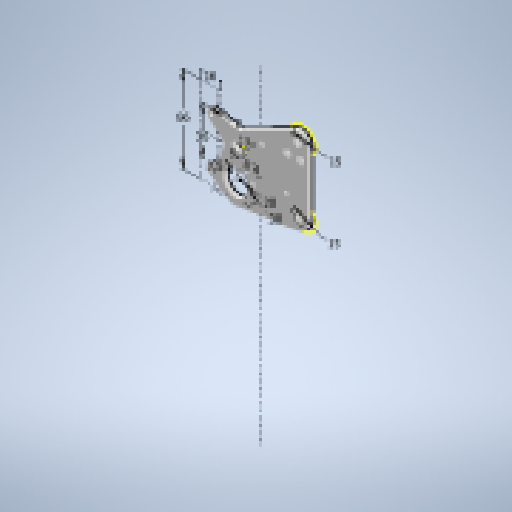
# Autodesk Inventor part: plate_3
Saved by Autodesk Inventor 2024 (Build 280153000, 153)
## iProperties
Created: 2026-02-08
Part Number: plate_3
Material: Generic
Document SubType Name: Modeling
Designer: SEMEN
Density: 1 g/cm^3
Appearance: Default
Author: SEMEN
Autodesk Inventor part; units mm, degrees
ref_plane "YZ Plane" through (0, 0, 0) normal (1, 0, 0) x (0, 1, 0)
ref_plane "XZ Plane" through (0, 0, 0) normal (0, 1, 0) x (-1, 0, 0)
ref_plane "XY Plane" through (0, 0, 0) normal (0, 0, 1) x (1, 0, 0)
sketch "Sketch1" plane through (0, 0, 0) normal (0, 0, 1) x (1, 0, 0)
  circle A0 centre (57.407, 53.064) radius 2.5 projected
  circle A1 centre (57.407, 53.064) radius 10 projected
  circle A2 centre (13.407, 27.6606) radius 2.5 projected
  circle A3 centre (13.407, 27.6606) radius 10 projected
  circle A4 centre (57.407, 2.2572) radius 2.5 projected
  circle A5 centre (57.407, 2.2572) radius 10 projected
  line L0 (25.407, -164.9104) -> (25.407, 85.0896) construction
  arc A6 (64.907, 53.064) -> (53.9811, 59.7359) centre (57.407, 53.064) ccw
  arc A7 (58.5116, -5.161) -> (64.907, 2.2572) centre (57.407, 2.2572) ccw
  line L1 (10.407, 27.6606) -> (16.407, 27.6606) construction
  line L2 (10.407, 25.0106) -> (16.407, 25.0106)
  line L3 (16.407, 30.3106) -> (10.407, 30.3106)
  arc A8 (10.407, 30.3106) -> (10.407, 25.0106) centre (10.407, 27.6606) ccw
  arc A9 (16.407, 25.0106) -> (16.407, 30.3106) centre (16.407, 27.6606) ccw
  circle A10 centre (10.407, 2.8412) radius 10
  arc A11 (-3.8238, 7.5832) -> (12.6162, -11.9952) centre (10.407, 2.8412) ccw
  line L4 (12.6162, -11.9952) -> (58.5116, -5.161)
  line L5 (53.9811, 59.7359) -> (8.8392, 36.5564)
  line L6 (64.907, 2.2572) -> (64.907, 53.064)
  line L7 (3.9198, 30.8219) -> (-3.8238, 7.5832)
  line L8 (-3.8238, 7.5832) -> (-11.5466, -15.5932) construction
  line L9 (12.6162, -11.9952) -> (-11.5466, -15.5932) construction
  line L10 (-11.5466, -15.5932) -> (31.917, 20.9033) construction
  line L11 (-8.093, 51.8526) -> (-8.093, -0.1388) construction
  circle A12 centre (-8.093, 38.8412) radius 3.5 construction
  circle A13 centre (-8.093, 2.8412) radius 3.5 construction
  line L12 (-20.593, 53.8412) -> (-4.593, 53.8412) construction
  line L13 (-4.593, 53.8412) -> (-4.593, -12.1588) construction
  line L14 (-4.593, -12.1588) -> (-20.593, -12.1588) construction
  line L15 (-20.593, -12.1588) -> (-20.593, 53.8412) construction
  line L16 (-20.593, 20.8412) -> (-4.593, 20.8412) construction
  line L17 (-2.413, 11.817) -> (-10.2687, 5.5829)
  line L18 (-10.2687, 0.0996) -> (1.0826, -8.9085)
  arc A14 (-4.593, -1.7035) -> (-4.0348, -1.2128) centre (-8.093, 2.8412) ccw
  arc A15 (-10.2687, 5.5829) -> (-10.2687, 0.0996) centre (-8.093, 2.8412) ccw
  line L19 (1.8905, 24.7319) -> (-10.4816, 36.2829)
  line L20 (-7.3703, 42.2658) -> (11.9978, 38.1783)
  arc A16 (-7.3703, 42.2658) -> (-10.4816, 36.2829) centre (-8.093, 38.8412) ccw
  point P0 (18.407, 14.782)
  point P1 (23.5514, 8.6555)
  dimension "d52" = 15
  dimension "d53" = 15
  dimension "d54" = 3
  dimension "d55" = 5.3
  dimension "d56" = 20
  dimension "d57" = 30
  dimension "d58" = 4
  dimension "d59" = 8
  dimension "d93" = 7
  dimension "d94" = 7
  dimension "d95" = 36
  dimension "d96" = 16
  dimension "d97" = 66
  dimension "d99" = 3.5
  constraints: 44 end point, 25 tangent, 20 point on circle, 11 centre point, 7 coincident, 7 point on line, 3 midpoint, 3 parallel, 2 collinear, 2 horizontal, 2 symmetric about line, 2 vertical, 1 concentric, 1 perpendicular, 2 other
  measures "d52" diameter of A6
  measures "d53" diameter of A7
  measures "d54" distance of A3.centre L1.end
  measures "d55" diameter of A9
  measures "d56" diameter of A10
  measures "d57" diameter of A11
  measures "d58" distance from line of L10 point (18.407, 14.782)
  measures "d59" horizontal distance of A10.centre point (18.407, 14.782)
  measures "d93" diameter of A12
  measures "d94" diameter of A13
  measures "d95" distance of point (-8.093, 2.841) point (-8.093, 38.841)
  measures "d96" distance of L12.start L12.end
  measures "d97" distance of L14.end L12.start
  measures "d99" radius of A15
extrude "Extrusion1" add sketch "Sketch1" along normal blind 4 contours A0 | L5 A6 L6 A1 | A1 L6 A5 L4 A11 L7 A3 L5 | L5 A3 L7 L19 A16 L20 | L6 A7 L4 A5 | A3 | L18 A15 L17 L7 A11 | A4 picked at (52.4239, 56.8921) picked at (55.6672, -3.7922)
sketch "Sketch2" plane through (0, 0, 4) normal (0, 0, 1) x (1, 0, 0)
  circle A0 centre (13.407, 27.6606) radius 2.5 projected
  circle A1 centre (57.407, 2.2572) radius 2.5 projected
  circle A2 centre (57.407, 53.064) radius 2.5 projected
  line L0 (10.407, 27.6606) -> (16.407, 27.6606) construction
  line L1 (10.407, 24.9106) -> (16.407, 24.9106)
  line L2 (16.407, 30.4106) -> (10.407, 30.4106)
  arc A3 (10.407, 30.4106) -> (10.407, 24.9106) centre (10.407, 27.6606) ccw
  arc A4 (16.407, 24.9106) -> (16.407, 30.4106) centre (16.407, 27.6606) ccw
  point P0 (0, 0)
  dimension "d25" = 3
  dimension "d26" = 5.5
  constraints: 8 end point, 4 point on circle, 4 tangent, 2 centre point, 1 horizontal, 1 midpoint, 1 parallel
  measures "d25" distance of A0.centre L0.end
  measures "d26" diameter of A4
hole "Hole2" at (57.407, 53.064, 4) at (57.407, 2.2572, 4) direction (0, 0, -1) diameter 5.5 end through all clearance for "Countersunk Head GOST 12876-67" size "M5" standard "GOST"
hole "Hole4" at (18.407, 14.782, 0) at (23.5514, 8.6555, 0) direction (0, 0, 1) diameter 3 end through all
sketch "Sketch6" plane through (0, 0, 0) normal (0, 0, -1) x (-1, 0, 0)
  circle A0 centre (-49.2903, 15.4803) radius 1.7 projected
  circle A1 centre (-30.2236, 38.1868) radius 1.7 projected
  point P0 (0, 0)
hole "Hole6" at (49.2903, 15.4803, 0) at (30.2236, 38.1868, 0) direction (0, 0, 1) diameter 3.4 end through all countersink diameter 6.6 countersink angle 90 clearance for "Countersunk Head GOST 12876-67" size "M3" standard "GOST"
sketch "Sketch7" plane through (0, 0, 4) normal (0, 0, 1) x (1, 0, 0)
  point P0 (0, 0)
  point P1 (49.6217, 42.3118)
  point P2 (59.6217, 42.3118)
hole "Hole7" at (59.6217, 42.3118, 4) at (49.6217, 42.3118, 4) direction (0, 0, -1) diameter 3.4 end through all countersink diameter 6.6 countersink angle 90 clearance for "Countersunk Head GOST 12876-67" size "M3" standard "GOST"
hole "Hole8" at (-8.093, 2.8412, 0) at (-8.093, 38.8412, 0) direction (0, 0, 1) diameter 3.4 end through all clearance for "Hex Head Bolt / Nut GOST 12876-67" size "M3" standard "GOST"
fillet "Fillet2" radius 5 3 edges at (-2.413, 11.817, 2) (1.8905, 24.7319, 2) (11.9978, 38.1783, 2)
body "Solid1"
